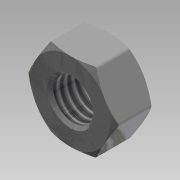
# Autodesk Inventor part: bed nut
Saved by Autodesk Inventor 2014 (Build 180170000, 170)
## iProperties
Created: 2016-03-31
Part Number: bed nut
Material: Stainless Steel
Document SubType Name: Modeling
Designer: admin
Density: 8.08 g/cm^3
Appearance: Semi-Polished
Author: admin
Autodesk Inventor part; units mm, degrees
ref_plane "YZ Plane" through (0, 0, 0) normal (1, 0, 0) x (0, 1, 0)
ref_plane "XZ Plane" through (0, 0, 0) normal (0, 1, 0) x (-1, 0, 0)
ref_plane "XY Plane" through (0, 0, 0) normal (0, 0, 1) x (1, 0, 0)
sketch "Sketch1" plane through (0, 0, 0) normal (0, 1, 0) x (-1, 0, 0)
  line L0 (3.7528, 6.5) -> (7.5056, 0)
  line L1 (7.5056, 0) -> (3.7528, -6.5)
  line L2 (3.7528, -6.5) -> (-3.7528, -6.5)
  line L3 (-3.7528, -6.5) -> (-7.5056, 0)
  line L4 (-7.5056, 0) -> (-3.7528, 6.5)
  line L5 (-3.7528, 6.5) -> (3.7528, 6.5)
  point P0 (0, 0)
  point P1 (0, 0)
  dimension "d0" = 6.5
  constraints: 12 end point, 1 coincident, 13 other
  measures "d0" distance from line of point (0, 0) L5
extrude "Extrusion1" add sketch "Sketch1" along normal blind 6.5
sketch "Sketch2" plane through (0, 6.5, 0) normal (0, 1, 0) x (1, 0, 0)
  point P0 (0, 0)
hole "Hole1" at (0, 6.5, 0) direction (0, -1, 0) diameter 6.647 depth 8 tip angle 118 thread size "M8x1.25" class "6H" standard "ISO Metric profile"
sketch "Sketch3" plane through (0, 6.5, 0) normal (0, 1, 0) x (1, 0, 0)
  circle A0 centre (0, 0) radius 3.3235 projected
  circle A1 centre (0, 0) radius 6.5
  circle A2 centre (0, 0) radius 29.8584
  constraints: 2 centre point, 2 coincident
extrude "Extrusion2" cut sketch "Sketch3" against normal blind 1 draft -60 contours A2
sketch "Sketch4" plane through (0, 0, 0) normal (0, -1, 0) x (1, 0, 0)
  circle A0 centre (0, 0) radius 3.3235 projected
  circle A1 centre (0, 0) radius 6.5
  circle A2 centre (0, 0) radius 18
  constraints: 2 centre point, 2 coincident
extrude "Extrusion3" cut sketch "Sketch4" against normal blind 1 draft -60 contours A2
fillet "Fillet1" radius 0.5 6 edges at (-7.5056, 3.25, 0) (-3.7528, 3.25, 6.5) (3.7528, 3.25, 6.5) (7.5056, 3.25, 0) (3.7528, 3.25, -6.5) (-3.7528, 3.25, -6.5)
chamfer "Chamfer1" distance 0.5 angle 45 2 edges at (0, 6.5, -3.3235) (0, 0, -3.3235)
body "Solid1"
